Autodesk Fusion 360 part; units mm, degrees
(part 2 of 2)
equation "d622 = base_thickness"
equation "d623 = taper_angle"
equation "d624 = base_height"
equation "d625 = length - 2 * endOverhang"
equation "d626 = base_thickness"
equation "d628 = base_thickness"
equation "d645 = 0.5 in * sqrt(2)"
equation "d646 = 0.5 in * sqrt(2)"
equation "stretcher_length = length - 2 * endOverhang - 2 * base_thickness"
equation "d696 = ( 0.5 * sqrt(2) ) * 1 in"
equation "d697 = d696"
equation "d700 = stretcher_width"
equation "d704 = stretcher_width"
equation "d710 = panel_width"
equation "d714 = panel_width"
